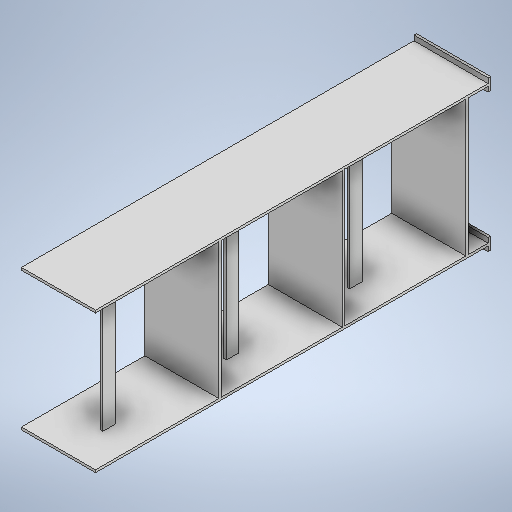
# Autodesk Inventor part: MoldStore
Saved by Autodesk Inventor 2025.1 (Build 291241000, 241)
## iProperties
Created: 2025-02-24
Part Number: MoldStore
Material: Generic
Document SubType Name: Modeling
Designer: yovan
Density: 1 g/cm^3
Appearance: Default
Author: yovan
Autodesk Inventor part; units mm, degrees
ref_plane "YZ Plane" through (0, 0, 0) normal (1, 0, 0) x (0, 1, 0)
ref_plane "XZ Plane" through (0, 0, 0) normal (0, 1, 0) x (-1, 0, 0)
ref_plane "XY Plane" through (0, 0, 0) normal (0, 0, 1) x (1, 0, 0)
sketch "Sketch1" plane through (0, 0, 0) normal (1, 0, 0) x (0, 1, 0)
  line L0 (0, 0) -> (10, 0)
  line L1 (10, 1600) -> (0, 1600)
  line L2 (0, 1600) -> (0, 10)
  line L3 (10, 100) -> (560, 100)
  line L4 (570, 100) -> (570, 90)
  line L5 (560, 90) -> (10, 90)
  line L6 (570, 0) -> (560, 0)
  line L7 (560, 1600) -> (570, 1600)
  line L8 (570, 1600) -> (570, 10)
  line L9 (10, 600) -> (560, 600)
  line L10 (10, 590) -> (560, 590)
  line L11 (10, 1100) -> (560, 1100)
  line L12 (10, 1090) -> (560, 1090)
  line L13 (540, 0) -> (590, 0)
  line L14 (590, 0) -> (590, 10)
  line L15 (540, 10) -> (540, 0)
  line L16 (-20, 0) -> (30, 0)
  line L17 (30, 0) -> (30, 10)
  line L18 (-20, 10) -> (-20, 0)
  line L19 (30, 10) -> (10, 10)
  line L20 (0, 10) -> (-20, 10)
  line L21 (590, 10) -> (570, 10)
  line L22 (560, 10) -> (540, 10)
  line L23 (560, 10) -> (560, 90)
  line L24 (10, 10) -> (10, 90)
  line L25 (10, 100) -> (10, 590)
  line L26 (560, 100) -> (560, 590)
  line L27 (560, 600) -> (560, 1090)
  line L28 (560, 1100) -> (560, 1600)
  line L29 (10, 600) -> (10, 1090)
  line L30 (10, 1100) -> (10, 1600)
  dimension "d0" = 10
  dimension "d1" = 1600
  dimension "d2" = 560
  dimension "d3" = 10
  dimension "d4" = 10
  dimension "d5" = 1600
  dimension "d6" = 50
  dimension "d7" = 10
  dimension "d8" = 50
  dimension "d9" = 10
  constraints: 62 end point, 31 perpendicular, 16 parallel, 5 horizontal
  measures "d0" distance of L1.end L1.start
  measures "d1" distance of L1.start L0.end
  measures "d2" distance of L3.start L4.start
  measures "d3" distance of L4.start L4.end
  measures "d4" distance of L7.start L7.end
  measures "d5" distance of L6.end L7.start
  measures "d6" distance of L15.start L14.end
  measures "d7" distance of L14.end L13.end
  measures "d8" distance of L18.start L17.end
  measures "d9" distance of L17.end L16.end
extrude "Extrusion1" add sketch "Sketch1" along normal blind 300
sketch "Sketch2" plane through (0, 10, 1600) normal (0, 1, 0) x (1, 0, 0)
  line L0 (0, 500) -> (200, 500)
  line L1 (200, 500) -> (200, 100)
  line L2 (200, 100) -> (0, 100)
  line L3 (0, 100) -> (0, 500)
  line L4 (200, 100) -> (180, 100)
  line L5 (180, 100) -> (180, 165)
  line L6 (180, 165) -> (200, 165)
  line L7 (200, 165) -> (200, 100)
  line L8 (180, 100) -> (0, 100)
  line L9 (0, 100) -> (0, 150)
  line L10 (0, 150) -> (180, 150)
  line L11 (180, 150) -> (180, 100)
  line L12 (180, 150) -> (170, 150)
  line L13 (170, 150) -> (170, 200)
  line L14 (170, 200) -> (180, 200)
  line L15 (180, 200) -> (180, 150)
  line L16 (0, 1000) -> (0, 510) projected
  line L17 (0, 1000) -> (180, 1000)
  line L18 (180, 1000) -> (180, 650)
  line L19 (180, 650) -> (0, 650)
  line L20 (0, 650) -> (0, 1000)
  line L21 (0, 1500) -> (180, 1500)
  line L22 (180, 1500) -> (180, 1150)
  line L23 (180, 1150) -> (0, 1150)
  line L24 (0, 1150) -> (0, 1500)
  line L25 (180, 650) -> (170, 650)
  line L26 (170, 650) -> (170, 700)
  line L27 (170, 700) -> (180, 700)
  line L28 (180, 700) -> (180, 650)
  line L29 (180, 1150) -> (170, 1150)
  line L30 (170, 1150) -> (170, 1200)
  line L31 (170, 1200) -> (180, 1200)
  line L32 (180, 1200) -> (180, 1150)
  point P0 (0, 1600)
  dimension "d12" = 200
  dimension "d13" = 400
  dimension "d14" = 20
  dimension "d15" = 65
  dimension "d16" = 180
  dimension "d17" = 50
  dimension "d18" = 10
  dimension "d19" = 50
  dimension "d20" = 180
  dimension "d21" = 350
  dimension "d22" = 180
  dimension "d23" = 350
  dimension "d24" = 10
  dimension "d25" = 50
  dimension "d26" = 10
  dimension "d27" = 50
  constraints: 64 end point, 16 parallel, 8 horizontal, 8 perpendicular
  measures "d12" distance of L1.end L2.end
  measures "d13" distance of L0.end L1.end
  measures "d14" distance of L5.end L6.end
  measures "d15" distance of L4.end L5.end
  measures "d16" distance of L9.end L10.end
  measures "d17" distance of L8.end L9.end
  measures "d18" distance of L13.end L14.end
  measures "d19" distance of L12.end L13.end
  measures "d20" distance of L18.end L19.end
  measures "d21" distance of L17.end L18.end
  measures "d22" distance of L22.end L23.end
  measures "d23" distance of L21.end L22.end
  measures "d24" distance of L26.end L27.end
  measures "d25" distance of L25.end L26.end
  measures "d26" distance of L30.end L31.end
  measures "d27" distance of L29.end L30.end
extrude "Extrusion2" add sketch "Sketch2" along normal blind 550 contours L13 L14 L15 L5 L10 | L26 L27 L18 L19 | L22 L23 L30 L31
body "Solid1"
